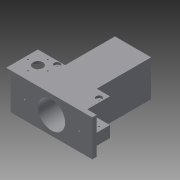
# Autodesk Inventor part: extruderBody
Saved by Autodesk Inventor 2015 SP2 (Build 190223200, 223)
## iProperties
Created: 2016-03-01
Part Number: extruderBody
Material: Generic
Document SubType Name: Modeling
Designer: marc
Density: 1 g/cm^3
Appearance: Default
Author: marc
Autodesk Inventor part; units mm, degrees
ref_plane "YZ Plane" through (0, 0, 0) normal (1, 0, 0) x (0, 1, 0)
ref_plane "XZ Plane" through (0, 0, 0) normal (0, 1, 0) x (-1, 0, 0)
ref_plane "XY Plane" through (0, 0, 0) normal (0, 0, 1) x (1, 0, 0)
sketch "Sketch4" plane through (0, 0, 0) normal (0, 1, 0) x (-1, 0, 0)
  line L0 (-90, 40) -> (90, 40)
  line L1 (90, 40) -> (90, -40)
  line L2 (90, -40) -> (-90, -40)
  line L3 (-90, -40) -> (-90, 40)
  line L4 (-90, 40) -> (90, -40) construction
  line L5 (90, 40) -> (-90, -40) construction
  point P0 (0, 0)
  dimension "width" = 80
  dimension "length" = 180
  constraints: 12 end point, 2 midpoint, 2 parallel, 1 horizontal, 1 perpendicular
  measures "width" distance of L2.end L0.start
  measures "length" distance of L1.end L2.end
extrude "Extrusion2" add sketch "Sketch4" along normal blind 180
sketch "Sketch18" plane through (0, 180, 0) normal (0, 1, 0) x (1, 0, 0)
  circle A0 centre (0, 0) radius 30
  dimension "syringeHole" = 60
  constraints: 1 centre point, 1 coincident
  measures "syringeHole" diameter of A0
extrude "Extrusion10" cut sketch "Sketch18" against normal through all
sketch "Sketch19" plane through (-90, 0, 40) normal (0, 0, 1) x (1, 0, 0)
  line L0 (180, 180) -> (130, 180)
  line L1 (130, 180) -> (130, 10)
  line L2 (130, 10) -> (180, 10)
  line L3 (180, 10) -> (180, 180)
  line L4 (0, 180) -> (50, 180)
  line L5 (50, 180) -> (50, 10)
  line L6 (50, 10) -> (0, 10)
  line L7 (0, 10) -> (0, 180)
  line L8 (90, 0) -> (90, 284.3953) construction
  line L9 (180, 0) -> (0, 0) construction
  dimension "flangethick" = 10
  dimension "flange" = 50
  constraints: 18 end point, 4 parallel, 2 horizontal, 2 perpendicular, 1 collinear, 1 vertical, 2 other
  measures "flangethick" distance between parallel lines of L9 L2
  measures "flange" distance between parallel lines of L3 L1
extrude "Extrusion11" cut sketch "Sketch19" against normal through all
sketch "Sketch20" plane through (-90, 0, 40) normal (0, 0, 1) x (1, 0, 0)
  line L0 (0, 0) -> (180, 0) projected
  line L1 (50, 0) -> (-10, 0)
  line L2 (-10, 0) -> (-10, 70)
  line L3 (-10, 70) -> (50, 70)
  line L4 (50, 70) -> (50, 0)
  line L5 (50, 180) -> (50, 10) projected
  point P0 (90, 0)
  dimension "motorSupportH" = 70
  dimension "motorSupportWidth" = 60
  constraints: 8 end point, 2 parallel, 1 collinear, 1 horizontal, 1 perpendicular, 1 point on line
  measures "motorSupportH" distance between parallel lines of L1 L3
  measures "motorSupportWidth" distance between parallel lines of L4 L2
extrude "Extrusion12" add sketch "Sketch20" against normal blind 5
sketch "Sketch23" plane through (0, 0, 0) normal (0, -1, 0) x (1, 0, 0)
  line L0 (122.132, 0) -> (-111.1675, 0) construction
  line L1 (0, -66.8528) -> (0, 59.8477) construction
  point P0 (0, 0)
  point P1 (60, 0)
  point P2 (-60, 0)
  dimension "flangehole" = 60
  constraints: 4 end point, 3 point on line, 1 horizontal, 1 symmetric about line, 1 vertical
  measures "flangehole" distance from line of point (60, 0) L1
hole "Hole2" at (60, 0, 0) at (-60, 0, 0) direction (0, 1, 0) diameter 4 end through all
sketch "Sketch24" plane through (-90, 0, 35) normal (0, 0, -1) x (-1, 0, 0)
  line L0 (-20, 18.0797) -> (-41.9203, 40) construction
  line L1 (-41.9203, 40) -> (-20, 61.9203) construction
  line L2 (-20, 61.9203) -> (1.9203, 40) construction
  line L3 (1.9203, 40) -> (-20, 18.0797) construction
  line L4 (-20, 106.0808) -> (-20, -9.0917) construction
  line L5 (10, 0) -> (10, 70) construction
  line L6 (-41.9203, 40) -> (1.9203, 40) construction
  line L7 (10, 70) -> (-50, 70) construction
  point P0 (-90, 0)
  dimension "motorHoleXoffset" = 30
  dimension "d74" = 31
  dimension "motorHoleYoffset" = 30
  constraints: 12 end point, 4 coincident, 2 parallel, 2 perpendicular, 2 point on line, 1 horizontal, 1 vertical
  measures "motorHoleXoffset" distance between parallel lines of L5 L4
  measures "d74" distance of L0.start L0.end
  measures "motorHoleYoffset" distance between parallel lines of L7 L6
hole "Hole3" at (-70, 61.9203, 35) at (-91.9203, 40, 35) at (-70, 18.0797, 35) at (-48.0797, 40, 35) direction (0, 0, 1) diameter 3 end through all
sketch "Sketch27" plane through (40, 10, 40) normal (0, 1, 0) x (1, 0, 0)
  line L0 (0, 0) -> (0, 80) projected
  line L1 (50, 0) -> (0, 0)
  line L2 (0, 0) -> (0, 25)
  line L3 (0, 25) -> (50, 25)
  line L4 (50, 25) -> (50, 0)
  line L5 (50, 80) -> (0, 80)
  line L6 (0, 80) -> (0, 55)
  line L7 (0, 55) -> (50, 55)
  line L8 (50, 55) -> (50, 80)
  line L9 (50, 80) -> (50, 0) projected
  line L10 (0, 80) -> (50, 80) projected
  point P0 (-40, 40)
  dimension "d93" = 30
  dimension "d94" = 25
  constraints: 16 end point, 4 parallel, 2 collinear, 2 horizontal, 2 perpendicular, 2 point on line
  measures "d93" distance between parallel lines of L3 L7
  measures "d94" distance between parallel lines of L1 L3
extrude "Extrusion15" add sketch "Sketch27" along normal blind 50 contours L0 L3 L4 L1 | L0 L5 L8 L7
sketch "Sketch28" plane through (90, 0, -40) normal (0, 0, -1) x (-1, 0, 0)
  line L0 (0, 0) -> (0, 60) projected
  line L1 (0, 60) -> (50, 60) projected
  line L2 (50, 180) -> (50, 60) projected
  point P0 (90, 0)
  point P1 (30, 45)
  dimension "d98" = 15
  dimension "drivenGearHoleOffsetX" = 20
  measures "d98" distance from line of L1 point (30, 45)
  measures "drivenGearHoleOffsetX" distance from line of point (30, 45) L2
hole "Hole4" at (60, 45, -40) direction (0, 0, 1) diameter 3 end through all
sketch "Sketch29" plane through (-90, 0, 35) normal (0, 0, -1) x (-1, 0, 0)
  circle A0 centre (-20, 40) radius 11
  line L0 (10, 0) -> (10, 70) projected
  line L1 (10, 70) -> (-50, 70) projected
  point P0 (-90, 0)
  point P1 (-29.1244, 70)
  dimension "motorShaftExit" = 22
  dimension "motorShaftXoffset" = 30
  dimension "motorShaftYoffset" = 30
  constraints: 1 centre point
  measures "motorShaftExit" diameter of A0
  measures "motorShaftXoffset" distance from line of L0 A0.centre
  measures "motorShaftYoffset" distance from line of L1 A0.centre
extrude "Extrusion16" cut sketch "Sketch29" against normal through all
sketch "Sketch31" plane through (90, 0, -40) normal (0, 0, -1) x (-1, 0, 0)
  circle A0 centre (30, 45) radius 1.5 projected
  circle A1 centre (30, 45) radius 6.5
  point P0 (90, 0)
  dimension "bearingOd" = 13
  constraints: 1 centre point, 1 coincident
  measures "bearingOd" diameter of A1
extrude "Extrusion17" cut sketch "Sketch31" against normal blind 5
sketch "Sketch32" plane through (-40, 180, 40) normal (0, 0, 1) x (1, 0, 0)
  circle A0 centre (100, -135) radius 1.5 projected
  circle A1 centre (100, -135) radius 6.5
  point P0 (40, -180)
  dimension "d114" = 13
  constraints: 1 centre point, 1 coincident
  measures "d114" diameter of A1
extrude "Extrusion18" cut sketch "Sketch32" against normal blind 5
sketch "Sketch36" plane through (-40, 180, 40) normal (0, 0, 1) x (1, 0, 0)
  line L0 (-60, -110) -> (0, -110) projected
  circle A0 centre (-10, -117.5) radius 7.5
  line L1 (-15.3033, -122.8033) -> (0, -138.1066)
  line L2 (0, -170) -> (0, -110) projected
  circle A1 centre (-10, -117.5) radius 2
  line L3 (-10, -110) -> (0, -110)
  point P0 (40, -180)
  dimension "d126" = 45
  dimension "d127" = 15
  dimension "idlerShaftOffsetX" = 10
  dimension "idlerShaftd" = 4
  constraints: 4 end point, 3 tangent, 2 centre point, 2 point on circle, 2 point on line, 1 coincident, 1 perpendicular
  measures "d126" angle of L2 L1
  measures "d127" diameter of A0
  measures "idlerShaftOffsetX" distance from line of L2 A0.centre
  measures "idlerShaftd" diameter of A1
extrude "Extrusion21" add sketch "Sketch36" against normal blind 63
sketch "Sketch37" plane through (-100, 70, 40) normal (0, 1, 0) x (1, 0, 0)
  line L0 (100, 40) -> (-34.5074, 40) construction
  line L1 (100, 40) -> (100, 230.6416) construction
  line L2 (60, 30) -> (40, 30)
  line L3 (40, 30) -> (40, 50)
  line L4 (40, 50) -> (60, 50)
  line L5 (60, 50) -> (60, 30)
  line L6 (60, 30) -> (40, 50) construction
  line L7 (40, 30) -> (60, 50) construction
  line L8 (60, 80) -> (60, 0) projected
  point P0 (50, 40)
  dimension "d132" = 20
  dimension "d133" = 20
  constraints: 16 end point, 2 horizontal, 2 midpoint, 2 parallel, 1 collinear, 1 perpendicular, 1 point on line, 1 vertical
  measures "d132" distance of L3.end L4.end
  measures "d133" distance of L2.end L3.end
extrude "Extrusion22" cut sketch "Sketch37" against normal up to surface (60 mm away)
sketch "Sketch39" plane through (-40, 180, -23) normal (0, 0, -1) x (-1, 0, 0)
  circle A0 centre (10, -117.5) radius 2
  circle A1 centre (10, -117.5) radius 2 projected
  point P0 (-40, -180)
  constraints: 2 concentric, 1 centre point
extrude "Extrusion23" cut sketch "Sketch39" against normal through all
sketch "Sketch40" plane through (-40, 180, 40) normal (0, 0, 1) x (1, 0, 0)
  circle A0 centre (-10, -117.5) radius 6.5
  circle A1 centre (-10, -117.5) radius 2 projected
  point P0 (40, -180)
  dimension "d138" = 13
  constraints: 1 centre point, 1 concentric
  measures "d138" diameter of A0
extrude "Extrusion24" cut sketch "Sketch40" against normal blind 5
sketch "Sketch41" plane through (90, 0, -40) normal (0, 0, -1) x (-1, 0, 0)
  line L0 (0, 60) -> (21, 60)
  line L1 (21, 60) -> (21, 10)
  line L2 (21, 10) -> (0, 10)
  line L3 (0, 10) -> (0, 60)
  line L4 (180, 0) -> (0, 0) projected
  point P0 (90, 0)
  dimension "d144" = 10
  dimension "d145" = 21
  constraints: 8 end point, 2 parallel, 1 horizontal, 1 perpendicular
  measures "d144" distance from line of L4 L2.end
  measures "d145" distance between parallel lines of L1 L3
extrude "Extrusion25" cut sketch "Sketch41" against normal through all
equation "\"d114\" = bearingOd"
equation "\"d115\" = bearingDepth"
equation "\"d138\" = bearingOd"
equation "\"d139\" = bearingDepth"
equation "\"d144\" = flangethick"
equation "\"d146\" = bearingDepth"
equation "\"bearingDepth\" = 5"
body "Solid2"
